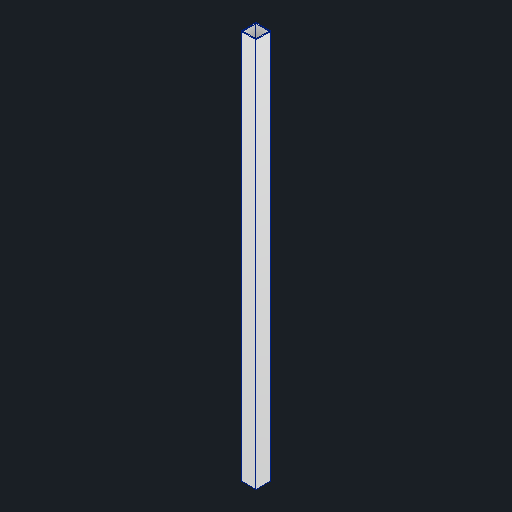
# Autodesk Inventor part: 64cmTube
Saved by Autodesk Inventor 2026.1 (Build 301233020, 233B)
## iProperties
Created: 2023-09-27
Part Number: 64cmTube
Material: Aluminum 6061
Document SubType Name: Modeling
Designer: Megan
Density: 2.7 g/cm^3
Appearance: Aluminum - Flat
Author: Megan
Autodesk Inventor part; units mm, degrees
ref_plane "YZ Plane" through (0, 0, 0) normal (1, 0, 0) x (0, 1, 0)
ref_plane "XZ Plane" through (0, 0, 0) normal (0, 1, 0) x (-1, 0, 0)
ref_plane "XY Plane" through (0, 0, 0) normal (0, 0, 1) x (1, 0, 0)
sketch "Sketch1" plane through (0, 0, 0) normal (0, 1, 0) x (-1, 0, 0)
  line L0 (12.7, 12.7) -> (12.7, -12.7)
  line L1 (12.7, -12.7) -> (-12.7, -12.7)
  line L2 (-12.7, -12.7) -> (-12.7, 12.7)
  line L3 (-12.7, 12.7) -> (12.7, 12.7)
  line L4 (12.7, 12.7) -> (-12.7, -12.7) construction
  line L5 (12.7, -12.7) -> (-12.7, 12.7) construction
  line L6 (11.1125, 11.1125) -> (11.1125, -11.1125)
  line L7 (11.1125, -11.1125) -> (-11.1125, -11.1125)
  line L8 (-11.1125, -11.1125) -> (-11.1125, 11.1125)
  line L9 (-11.1125, 11.1125) -> (11.1125, 11.1125)
  line L10 (11.1125, 11.1125) -> (-11.1125, -11.1125) construction
  line L11 (11.1125, -11.1125) -> (-11.1125, 11.1125) construction
  point P0 (0, 0)
  dimension "d0" = 25.4
  dimension "d1" = 25.4
  dimension "d2" = 1.5875
  dimension "d3" = 1.5875
  constraints: 24 end point, 4 midpoint, 4 parallel, 2 perpendicular, 2 vertical
  measures "d0" distance of L0.start L0.end
  measures "d1" distance of L0.end L1.end
  measures "d2" distance between parallel lines of L0 L6
  measures "d3" distance between parallel lines of L1 L7
extrude "Extrusion1" add sketch "Sketch1" along normal blind 660.4
body "Solid1"
